holderTop_v22 (Autodesk Fusion 360 design; units mm, degrees)
Autodesk Fusion 360 part; units mm, degrees
note: some values were not read from the file. Set by a fixed rule: the direction of a hole.
sketch "Sketch1" plane through (0, 0, 0) normal (0, 0, 1) x (1, 0, 0)
  circle A0 centre (0, 0) radius 25.4
  circle A1 centre (0, 0) radius 22.225 construction
  line L0 (0, 0) -> (0, 25.4) construction
  circle A2 centre (0, 0) radius 15.0812 construction
  point P0 (0, 22.225)
  point P1 (0, 15.0812)
  dimension "d1" = 50.8
  dimension "d2" = 44.45
  dimension "d3" = 30.1625
  constraint coincident A0.centre A1.centre
  constraint coincident A0 L0.end
  constraint vertical L0
  constraint coincident A1 P0
  constraint coincident L0 P0
  constraint coincident A2 P1
  constraint coincident L0 P1
  measures "d1" diameter of A0
  measures "d2" diameter of A1
  measures "d3" diameter of A2
extrude "Extrude1" add sketch "Sketch1" along normal blind 6.35
hole "Hole1" at (0, 22.225, 0) direction (0, 0, 1) diameter 4.4958 depth 6.35 tip angle 118
hole "Hole2" at (0, 15.0812, 0) direction (0, 0, 1) diameter 3.7973 depth 6.35 tip angle 118
pattern_circular "C-Pattern1" count 3 over 360 about axis through (0, 0, 0) along (0, 0, 1) of "Hole1"
pattern_circular "C-Pattern2" count 3 over 360 about axis through (0, 0, 0) along (0, 0, 1) of "Hole2"
hole "Hole3" at (0, 0, 0) direction (0, 0, 1) diameter 2.2708 depth 6.35 tip angle 180
thread "Thread1" "ANSI Unified Screw Threads 0.112(#4) 4-40 UNC 2B"
